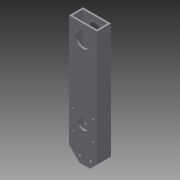
# Autodesk Inventor part: SuperStructure
Saved by Autodesk Inventor 2013 (Build 170138000, 138)
## iProperties
Created: 2014-01-20
Part Number: SuperStructure
Material: Generic
Document SubType Name: Modeling
Designer: RobertB
Density: 1 g/cm^3
Author: RobertB
Autodesk Inventor part; units mm, degrees
ref_plane "YZ Plane" through (0, 0, 0) normal (1, 0, 0) x (0, 1, 0)
ref_plane "XZ Plane" through (0, 0, 0) normal (0, 1, 0) x (-1, 0, 0)
ref_plane "XY Plane" through (0, 0, 0) normal (0, 0, 1) x (1, 0, 0)
sketch "Sketch1" plane through (0, 0, 0) normal (0, 1, 0) x (-1, 0, 0)
  line L0 (25.4, 12.7) -> (-25.4, 12.7)
  line L1 (-25.4, 12.7) -> (-25.4, -12.7)
  line L2 (-25.4, -12.7) -> (25.4, -12.7)
  line L3 (25.4, -12.7) -> (25.4, 12.7)
  line L4 (25.4, 12.7) -> (-25.4, -12.7) construction
  line L5 (-25.4, 12.7) -> (25.4, -12.7) construction
  line L6 (22.225, 9.525) -> (-22.225, 9.525)
  line L7 (-22.225, 9.525) -> (-22.225, -9.525)
  line L8 (-22.225, -9.525) -> (22.225, -9.525)
  line L9 (22.225, -9.525) -> (22.225, 9.525)
  line L10 (22.225, 9.525) -> (-22.225, -9.525) construction
  line L11 (-22.225, 9.525) -> (22.225, -9.525) construction
  point P0 (0, 0)
  dimension "d0" = 50.8
  dimension "d1" = 25.4
  dimension "d2" = 44.45
  dimension "d3" = 19.05
  constraints: 24 end point, 4 midpoint, 4 parallel, 2 horizontal, 2 perpendicular
  measures "d0" distance of L2.end L1.end
  measures "d1" distance of L1.end L0.end
  measures "d2" distance of L8.end L7.end
  measures "d3" distance of L7.end L6.end
extrude "Extrusion1" add sketch "Sketch1" along normal blind 228.6
sketch "Sketch2" plane through (-25.4, 0, 12.7) normal (0, 0, 1) x (1, 0, 0)
  line L0 (50.8, 0) -> (50.8, 228.6) projected
  line L1 (0, 228.6) -> (50.8, 228.6) projected
  line L2 (0, 0) -> (0, 228.6) projected
  line L3 (25.4, 228.6) -> (25.4, 203.2)
  circle A0 centre (25.4, 203.2) radius 6.35
  line L4 (25.4, 203.2) -> (25.4, 25.4)
  line L5 (25.4, 203.2) -> (203.2, 203.2) construction
  line L6 (25.4, 25.4) -> (50.8, 25.4)
  line L7 (50.8, 25.4) -> (0, 25.4)
  line L8 (25.4, 25.4) -> (25.4, 19.05)
  line L9 (25.4, 25.4) -> (31.75, 25.4) construction
  line L10 (25.4, 19.05) -> (50.8, 19.05)
  line L11 (25.4, 19.05) -> (0, 19.05)
  line L12 (25.4, 19.05) -> (38.1, 19.05)
  line L13 (38.1, 19.05) -> (19.05, 19.05)
  circle A1 centre (38.1, 19.05) radius 2.54
  circle A2 centre (19.05, 19.05) radius 2.54
  point P0 (25.4, 0)
  dimension "d6" = 25.4
  dimension "d7" = 12.7
  dimension "d8" = 177.8
  dimension "d9" = 90
  dimension "d10" = 6.35
  dimension "d11" = 90
  dimension "d12" = 12.7
  dimension "d13" = 19.05
  dimension "d14" = 0
  dimension "d15" = 5.08
  dimension "d16" = 5.08
  constraints: 22 end point, 6 perpendicular, 4 point on line, 3 centre point, 3 coincident, 3 collinear, 2 horizontal, 2 midpoint, 1 parallel
  measures "d6" distance of L3.start L3.end
  measures "d7" diameter of A0
  measures "d8" distance of L4.start L4.end
  measures "d9" angle of L4 L5
  measures "d10" distance of L4.end L8.end
  measures "d11" angle of L8 L9
  measures "d12" distance of L8.end L12.end
  measures "d13" distance of L12.end L13.end
  measures "d14" distance between parallel lines of L13 L12
  measures "d15" diameter of A1
  measures "d16" diameter of A2
extrude "Extrusion2" cut sketch "Sketch2" against normal blind 228.6 contours A1 L10 | L10 A1 | L4 L3 A0 | A0 L3 L4 | A2 L11 | L11 A2
sketch "Sketch3" plane through (0, 0, 0) normal (0, -1, 0) x (1, 0, 0)
  line L0 (-22.225, -9.525) -> (-22.225, 9.525) projected
  line L1 (-22.225, 9.525) -> (22.225, 9.525) projected
  line L2 (22.225, 9.525) -> (22.225, -9.525) projected
  line L3 (22.225, -9.525) -> (-22.225, -9.525) projected
  line L4 (-25.4, 12.7) -> (25.4, 12.7) projected
  line L5 (-25.4, -12.7) -> (-25.4, 12.7) projected
  line L6 (25.4, -12.7) -> (-25.4, -12.7) projected
  line L7 (25.4, 12.7) -> (25.4, -12.7) projected
  point P0 (0, 0)
extrude "Extrusion3" cut sketch "Sketch3" against normal blind 6.35
sketch "Sketch4" plane through (-25.4, 228.6, 12.7) normal (0, 0, 1) x (1, 0, 0)
  line L0 (0, -222.25) -> (50.8, -222.25) projected
  line L1 (50.8, -222.25) -> (50.8, 0) projected
  line L2 (0, -222.25) -> (0, 0) projected
  line L3 (0, -209.55) -> (12.7, -222.25)
  line L4 (50.8, -209.55) -> (38.1, -222.25)
  point P0 (25.4, -228.6)
  constraints: 4 end point, 4 point on line, 1 perpendicular
extrude "Extrusion4" cut sketch "Sketch4" against normal blind 635
sketch "Sketch5" plane through (-25.4, 228.6, 12.7) normal (0, 0, 1) x (1, 0, 0)
  line L0 (0, -209.55) -> (12.7, -222.25) projected
  line L1 (12.7, -222.25) -> (38.1, -222.25) projected
  line L2 (38.1, -222.25) -> (50.8, -209.55) projected
  line L3 (0, -209.55) -> (0, 0) projected
  line L4 (19.05, -222.25) -> (0, -203.2)
  point P0 (25.4, -228.6)
  constraints: 2 end point, 2 point on line, 1 perpendicular
extrude "Extrusion5" cut sketch "Sketch5" against normal blind 635
sketch "Sketch6" plane through (-25.4, 228.6, 12.7) normal (0, 0, 1) x (1, 0, 0)
  line L0 (19.05, -222.25) -> (38.1, -222.25) projected
  line L1 (38.1, -222.25) -> (50.8, -209.55) projected
  line L2 (0, -203.2) -> (0, 0) projected
  line L3 (25.4, -222.25) -> (25.4, -158.75)
  line L4 (25.4, -222.25) -> (88.9, -222.25) construction
  circle A0 centre (25.4, -158.75) radius 9.525
  line L5 (25.4, -158.75) -> (43.3605, -140.7895)
  line L6 (25.4, -158.75) -> (50.8, -158.75) construction
  line L7 (43.3605, -140.7895) -> (7.4395, -176.7105)
  line L8 (7.4395, -176.7105) -> (43.3605, -176.7105)
  line L9 (43.3605, -176.7105) -> (43.3605, -140.7895)
  line L10 (43.3605, -140.7895) -> (7.4395, -140.7895)
  line L11 (7.4395, -140.7895) -> (7.4395, -176.7105)
  circle A1 centre (43.3605, -140.7895) radius 2.032
  circle A2 centre (7.4395, -140.7895) radius 2.032
  circle A3 centre (7.4395, -176.7105) radius 2.032
  circle A4 centre (43.3605, -176.7105) radius 2.032
  point P0 (25.4, -228.6)
  dimension "d25" = 63.5
  dimension "d26" = 90
  dimension "d27" = 19.05
  dimension "d28" = 25.4
  dimension "d29" = 45
  dimension "d30" = 50.8
  dimension "d31" = 4.064
  dimension "d32" = 4.064
  dimension "d33" = 4.064
  dimension "d34" = 4.064
  constraints: 18 end point, 5 centre point, 5 coincident, 4 parallel, 3 horizontal, 2 equal length, 1 collinear, 1 perpendicular, 1 point on line
  measures "d25" distance of L3.start L3.end
  measures "d26" angle of L4 L3
  measures "d27" diameter of A0
  measures "d28" distance of L5.start L5.end
  measures "d29" angle of L6 L5
  measures "d30" distance of L5.end L7.end
  measures "d31" diameter of A1
  measures "d32" diameter of A2
  measures "d33" diameter of A3
  measures "d34" diameter of A4
extrude "Extrusion6" cut sketch "Sketch6" against normal blind 635 contours A0 L7 L3 | L3 L5 A0 | A3 L11 L8 | L8 L7 A3 | A4 L9 L8 | L8 L9 A4 | L7 A0 L5 | L11 A3 L7 | A2 L10 L11 | L11 L10 A2 | A1 L5 L9 | L9 L10 A1 | A1 L10 L5
sketch "Sketch7" plane through (-25.4, 228.6, 12.7) normal (0, 0, 1) x (1, 0, 0)
  circle A0 centre (25.4, -25.4) radius 6.35 projected
  circle A1 centre (25.4, -25.4) radius 14.2875
  point P0 (25.4, -228.6)
  dimension "d37" = 28.575
  constraints: 1 centre point, 1 coincident
  measures "d37" diameter of A1
extrude "Extrusion7" cut sketch "Sketch7" against normal blind 635
body "Solid1"
